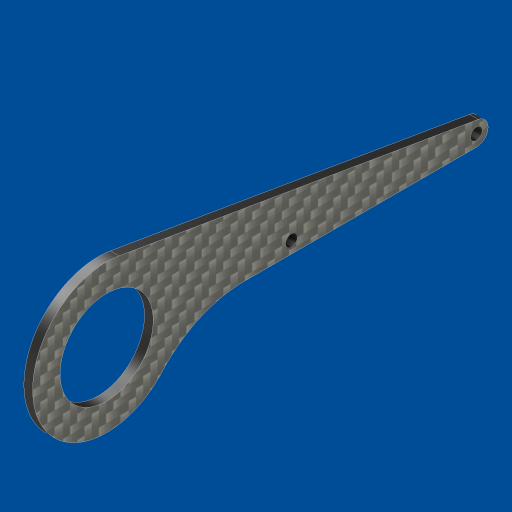
# Autodesk Inventor part: linkPanel
Saved by Autodesk Inventor 2023 (Build 270158030, 158C)
## iProperties
Created: 2023-03-03
Part Number: linkPanel
Material: CFRP
Document SubType Name: Modeling
Designer: kumpu
Density: 1.43 g/cm^3
Appearance: Glossy - Black
Author: kumpu
Autodesk Inventor part; units mm, degrees
ref_plane "YZ Plane" through (0, 0, 0) normal (1, 0, 0) x (0, 1, 0)
ref_plane "XZ Plane" through (0, 0, 0) normal (0, 1, 0) x (-1, 0, 0)
ref_plane "XY Plane" through (0, 0, 0) normal (0, 0, 1) x (1, 0, 0)
sketch "Sketch1" plane through (0, 0, 0) normal (1, 0, 0) x (0, 1, 0)
  line L0 (25.0368, -4.28) -> (3.9428, -127.674)
  arc A0 (-4, -127) -> (3.9428, -127.674) centre (0, -127) ccw
  arc A1 (25.0368, -4.28) -> (-16.84, -19.0151) centre (0, 0) ccw
  line L1 (0, 0) -> (0, -127) construction
  circle A2 centre (0, 0) radius 16
  circle A3 centre (0, -127) radius 2
  circle A4 centre (0, -63.5) radius 2
  line L2 (-4, -127) -> (-4, -47.5378)
  arc A5 (-4, -47.5378) -> (-16.84, -19.0151) centre (-42.1, -47.5378) ccw
  dimension "d0" = 32
  dimension "d1" = 127
  dimension "d2" = 4
  dimension "d3" = 25.4
  dimension "d4" = 4
  dimension "d7" = 63.5
  dimension "d14" = 38.1
  constraints: 6 centre point, 6 end point, 6 point on circle, 5 tangent, 3 coincident, 3 vertical, 2 other
  measures "d0" diameter of A2
  measures "d1" distance of L1.start L1.end
  measures "d2" radius of A0
  measures "d3" radius of A1
  measures "d4" diameter of A3
  measures "d7" distance of A3.centre A4.centre
  measures "d14" radius of A5
extrude "Extrusion1" add sketch "Sketch1" along normal blind 3
body "Solid1"
